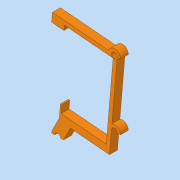
# Autodesk Inventor part: DriveBatteryHolder
Saved by Autodesk Inventor 2017 (Build 210142000, 142)
## iProperties
Created: 2018-01-30
Part Number: DriveBatteryHolder
Material: ABS Plastic
Document SubType Name: Modeling
Designer: Derek Wider
Density: 1.06 g/cm^3
Appearance: Orange
Author: Derek Wider
Autodesk Inventor part; units mm, degrees
ref_plane "YZ Plane" through (0, 0, 0) normal (1, 0, 0) x (0, 1, 0)
ref_plane "XZ Plane" through (0, 0, 0) normal (0, 1, 0) x (-1, 0, 0)
ref_plane "XY Plane" through (0, 0, 0) normal (0, 0, 1) x (1, 0, 0)
sketch "Sketch1" plane through (0, 0, 0) normal (0, 0, 1) x (1, 0, 0)
  arc A0 (1.905, 0) -> (-1.905, 0) centre (0, 0) ccw
  arc A1 (38.2001, 20.955) -> (34.3974, 21.121) centre (36.2951, 20.955) ccw
  arc A2 (38.2001, 62.865) -> (35.968, 60.9883) centre (36.2951, 62.865) ccw
  line L0 (31.0979, 11.275) -> (2.2082, 13.8025)
  line L1 (31.0979, 11.275) -> (60.0979, 11.275) construction
  line L2 (31.0979, 11.275) -> (35.4557, 61.0847)
  line L3 (35.4557, 61.0847) -> (4.305, 63.81)
  line L4 (-3.2733, 67.0227) -> (32.0141, 63.9355)
  line L5 (37.9446, 61.6656) -> (33.1202, 6.5228)
  line L6 (33.1202, 6.5228) -> (8.1809, 8.7047)
  arc A3 (40.1051, 20.955) -> (34.6849, 24.408) centre (36.2951, 20.955) ccw
  line L7 (40.1051, 20.955) -> (38.2001, 20.955)
  arc A4 (38.2001, 20.955) -> (34.3974, 21.121) centre (36.2951, 20.955) ccw
  arc A5 (40.1051, 62.865) -> (33.5702, 65.5278) centre (36.2951, 62.865) ccw
  line L8 (32.0141, 63.9355) -> (33.5702, 65.5278)
  line L9 (35.968, 60.9883) -> (36.0336, 60.9883)
  line L10 (36.0336, 60.9883) -> (37.9446, 61.6656)
  line L11 (38.2001, 62.865) -> (40.1051, 62.865)
  arc A6 (-3.4049, 1.7097) -> (-3.81, 0) centre (0, 0) ccw
  line L12 (-1.905, 0) -> (-3.81, 0)
  line L13 (1.905, 0) -> (3.81, 0)
  line L14 (1.0757, 10.6327) -> (-3.4049, 1.7097)
  line L15 (3.81, 0) -> (8.1809, 8.7047)
  line L16 (4.0283, 60.6471) -> (-3.7714, 61.3295)
  line L17 (2.651, 18.8631) -> (1.8023, 18.9374)
  line L18 (4.305, 63.81) -> (4.0283, 60.6471)
  line L19 (2.651, 18.8631) -> (2.2082, 13.8025)
  line L20 (1.0757, 10.6327) -> (1.8023, 18.9374)
  line L21 (-3.7714, 61.3295) -> (-3.2733, 67.0227)
  dimension "d0" = 3.81
  dimension "d1" = 3.81
  dimension "d2" = 3.81
  dimension "d3" = 41.91
  dimension "d4" = 41.91
  dimension "d5" = 120
  dimension "d6" = 185
  dimension "d7" = 29
  dimension "d8" = 50
  dimension "d9" = 2.54
  dimension "d10" = 7.62
  dimension "d11" = 3.81
  dimension "d12" = 6.35
  dimension "d13" = 7.62
  dimension "d14" = 5.08
  dimension "d15" = 3.175
  constraints: 44 end point, 14 point on circle, 7 centre point, 7 parallel, 6 perpendicular, 4 coincident, 4 horizontal, 4 point on line, 3 tangent, 1 concentric, 1 equal length, 1 horizontal alignment, 1 vertical alignment
  measures "d0" diameter of A0
  measures "d1" diameter of A1
  measures "d2" diameter of A2
  measures "d3" distance of A1.centre A2.centre
  measures "d4" distance of point (0, 0) A1.centre
  measures "d7" distance of L0.start L0.end
  measures "d8" distance of L0.start L2.end
  measures "d9" distance between parallel lines of L3 L4
  measures "d10" diameter of A5
  measures "d11" radius of A3
  measures "d12" distance of L5.start L4.end
  measures "d13" diameter of A6
  measures "d14" distance from line of L0.end L17
  measures "d15" distance between parallel lines of L16 L3
extrude "Extrusion1" add sketch "Sketch1" along normal blind 5.08
body "Solid1"
